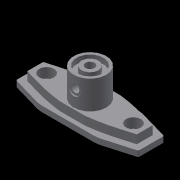
# Autodesk Inventor part: SpineConnector
Saved by Autodesk Inventor 2015 SP1 (Build 190203100, 203)
## iProperties
Created: 2014-12-04
Part Number: SpineConnector
Material: Generic
Document SubType Name: Modeling
Designer: Val
Density: 1 g/cm^3
Appearance: Default
Mass: 23.826 g
Surface Area: 97.027 cm^2
Volume: 23.826 cm^3
RuleStatus: InUse
BeforeDocSave0: UpdateBoundingBox
CX: 86.24 mm
CY: 31.00 mm
CZ: 30.00 mm
Author: Val
Autodesk Inventor part; units mm, degrees
note: some values were not read from the file. Chosen so that the rebuilt part matches the saved one: sketch regions of "BaseLayer2Feature"; sketch regions of "BaseLayer3Feature".
ref_plane "YZ Plane" through (0, 0, 0) normal (1, 0, 0) x (0, 1, 0)
ref_plane "XZ Plane" through (0, 0, 0) normal (0, 1, 0) x (-1, 0, 0)
sketch "Base" plane through (0, 0, 0) normal (0, 0, 1) x (1, 0, 0)
  circle A0 centre (-30.619, 0) radius 3.25
  circle A1 centre (0, 0) radius 3.25
  circle A2 centre (0, 0) radius 9.5
  circle A3 centre (0, 0) radius 11.5
  circle A4 centre (0, 0) radius 6
  arc A5 (-9, 12.5) -> (-29.4881, 8.2332) centre (6.3563, -112.5607) ccw
  circle A6 centre (-30.619, 0) radius 5.25
  line L0 (0, 12.5) -> (-9, 12.5)
  line L1 (-38.619, 5.6106) -> (-38.619, 0)
  line L2 (-43.119, 9) -> (-43.119, 0)
  line L3 (-43.119, 9) -> (-21.9739, 15.0735)
  line L4 (0, 15.5) -> (-18.5, 15.5)
  circle A7 centre (0, 0) radius 14.25
  line L5 (-38.619, 5.6106) -> (-29.4881, 8.2332)
  line L6 (-21.9739, 15.0735) -> (-18.5, 15.5)
  line L7 (0, -157.585) -> (0, 157.585) construction
  line L8 (-43.119, 0) -> (0, 0) construction
  line L9 (0, 15.5) -> (0, 0) construction
  arc A8 (-29.4881, -8.2332) -> (-9, -12.5) centre (6.3563, 112.5607) ccw
  line L10 (0, -12.5) -> (-9, -12.5)
  line L11 (-38.619, -5.6106) -> (-38.619, 0)
  line L12 (-43.119, -9) -> (-43.119, 0)
  line L13 (-43.119, -9) -> (-21.9739, -15.0735)
  line L14 (0, -15.5) -> (-18.5, -15.5)
  line L15 (-38.619, -5.6106) -> (-29.4881, -8.2332)
  line L16 (-21.9739, -15.0735) -> (-18.5, -15.5)
  circle A9 centre (30.619, 0) radius 3.25
  arc A10 (29.4881, 8.2332) -> (9, 12.5) centre (-6.3563, -112.5607) ccw
  circle A11 centre (30.619, 0) radius 5.25
  line L17 (0, 12.5) -> (9, 12.5)
  line L18 (38.619, 5.6106) -> (38.619, 0)
  line L19 (43.119, 9) -> (43.119, 0)
  line L20 (43.119, 9) -> (21.9739, 15.0735)
  line L21 (0, 15.5) -> (18.5, 15.5)
  line L22 (38.619, 5.6106) -> (29.4881, 8.2332)
  line L23 (21.9739, 15.0735) -> (18.5, 15.5)
  line L24 (43.119, -9) -> (43.119, 0)
  line L25 (43.119, -9) -> (21.9739, -15.0735)
  line L26 (21.9739, -15.0735) -> (18.5, -15.5)
  line L27 (0, -15.5) -> (18.5, -15.5)
  line L28 (0, -12.5) -> (9, -12.5)
  arc A12 (9, -12.5) -> (29.4881, -8.2332) centre (-6.3563, 112.5607) ccw
  line L29 (38.619, -5.6106) -> (29.4881, -8.2332)
  line L30 (38.619, -5.6106) -> (38.619, 0)
  dimension "d15" = 6.5
  dimension "d16" = 12
  dimension "d17" = 19
  dimension "d18" = 23
  dimension "d19" = 28.5
  dimension "d20" = 18.5
  dimension "d21" = 3.5
  dimension "d22" = 22
  dimension "d23" = 9
  dimension "d26" = 4.5
  dimension "d27" = 4.5
  dimension "d28" = 126
  dimension "d29" = 9
  dimension "d30" = 8
  dimension "d31" = 6.5
  dimension "d32" = 10.5
  dimension "d33" = 173
  dimension "d34" = 3
  dimension "d35" = 9.5
  dimension "d36" = 15.5
  constraints: 60 end point, 28 symmetric about line, 13 centre point, 8 point on circle, 5 concentric, 4 point on line, 3 horizontal, 3 vertical, 1 parallel, 5 other
  measures "d15" diameter of A1
  measures "d16" diameter of A4
  measures "d17" diameter of A2
  measures "d18" diameter of A3
  measures "d19" diameter of A7
  measures "d20" distance of L4.start L4.end
  measures "d21" distance of L3.end L4.end
  measures "d22" distance of L2.start L3.end
  measures "d23" distance of L2.start L2.end
  measures "d26" distance between parallel lines of L2 L1
  measures "d27" distance between parallel lines of L3 L5
  measures "d28" radius of A5
  measures "d29" distance of L0.start L0.end
  measures "d30" distance of L1.end A0.centre
  measures "d31" diameter of A0
  measures "d32" diameter of A6
  measures "d33" angle of L4 L6
  measures "d34" distance between parallel lines of L4 L0
  measures "d35" distance of L1.start L5.end
  measures "d36" distance of A1.centre L4.start
extrude "BaseLayer1Feature" add sketch "Base" along normal blind 3 contours A6 | A11
extrude "BaseLayer2Feature" add sketch "Base" along normal blind 10 contours A2 | A3 | A4 | L0 A7 L10 A8 L15 L11 L1 L5 A5 | L0 L17 A7 L28 L10 | L17 A10 L22 L18 L30 L29 A12 L28 A7
extrude "BaseLayer3Feature" add sketch "Base" along normal blind 4 contours A3 | A7 L17 L0 | L0 L17 A7 L28 L10 | L10 L28 A7 | L3 L6 L4 L21 L23 L20 L19 L24 L25 L26 L27 L14 L16 L13 L12 L2
extrude "SpineLinkMountFeature" add sketch "Base" along normal blind 30 contours A3 | A4
ref_plane "SpineLinkMountCountersinkPlane" through (0, 0, 26) normal (0, 0, 1) x (1, 0, 0)
extrude "SpineLinkMountCountresinkFeature" add sketch "Base" along normal up to surface (26 mm away) contours A2
fillet "OutsideSmallFilletsFeature" radius 1 4 edges at (-43.119, 9, 2) (-43.119, -9, 2) (43.119, 9, 2) (43.119, -9, 2)
fillet "OutsideLargeFilletsFeature" radius 2 8 edges at (-21.9739, 15.0735, 2) (-18.5, 15.5, 2) (18.5, 15.5, 2) (21.9739, 15.0735, 2) (-21.9739, -15.0735, 2) (-18.5, -15.5, 2) (18.5, -15.5, 2) (21.9739, -15.0735, 2)
sketch "SpineCoreHole" plane through (-9, -12.5, 10) normal (0, -1, 0) x (1, 0, 0)
  circle A0 centre (9, 11.5) radius 2.5
  line L0 (20.5, 20) -> (-2.5, 20) construction
  line L1 (0, 0) -> (18, 0) construction
  line L2 (9, 20) -> (9, 0) construction
  dimension "d57" = 5
  dimension "d58" = 8.5
  constraints: 2 end point, 2 midpoint, 1 centre point, 1 point on line
  measures "d57" diameter of A0
  measures "d58" distance from line of L0 A0.centre
hole "SpineCoreHoleFeature" at (0, -12.5, 21.5) direction (0, 1, 0) diameter 6 end through all counterbore diameter 9 counterbore depth 2
